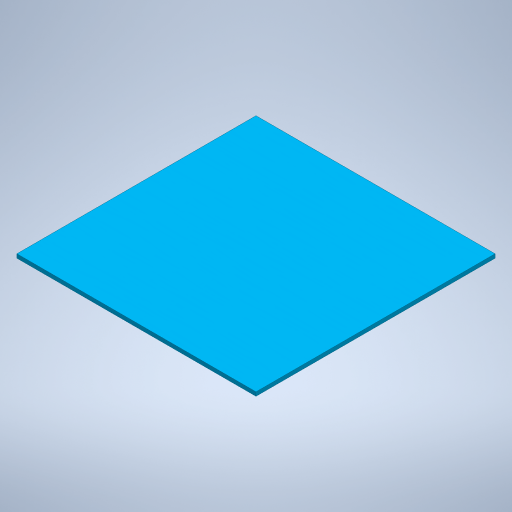
# Autodesk Inventor part: Lamina centelladora
Saved by Autodesk Inventor 2024.2 (Build 282272000, 272)
## iProperties
Created: 2025-06-13
Part Number: Lamina centelladora
Material: Plástico PMMA
Document SubType Name: Modeling
Designer: jd.castellanosq
Density: 1.188 g/cm^3
Appearance: Azul celeste medio
Author: jd.castellanosq
Autodesk Inventor part; units mm, degrees
ref_plane "YZ Plane" through (0, 0, 0) normal (1, 0, 0) x (0, 1, 0)
ref_plane "XZ Plane" through (0, 0, 0) normal (0, 1, 0) x (-1, 0, 0)
ref_plane "XY Plane" through (0, 0, 0) normal (0, 0, 1) x (1, 0, 0)
sketch "Boceto1" plane through (0, 0, 0) normal (0, 0, 1) x (1, 0, 0)
  line L0 (-305, 305) -> (305, 305)
  line L1 (305, 305) -> (305, -305)
  line L2 (305, -305) -> (-305, -305)
  line L3 (-305, -305) -> (-305, 305)
  point P0 (0, 0)
  point P1 (0, 305)
  point P2 (305, 0)
  dimension "d0" = 610
  dimension "d1" = 610
  constraints: 8 end point, 2 midpoint, 2 parallel, 1 horizontal, 1 horizontal alignment, 1 perpendicular, 1 vertical alignment
  measures "d0" distance of L0.start L0.end
  measures "d1" distance of L0.end L1.end
extrude "Extrusión1" add sketch "Boceto1" along normal blind 10
